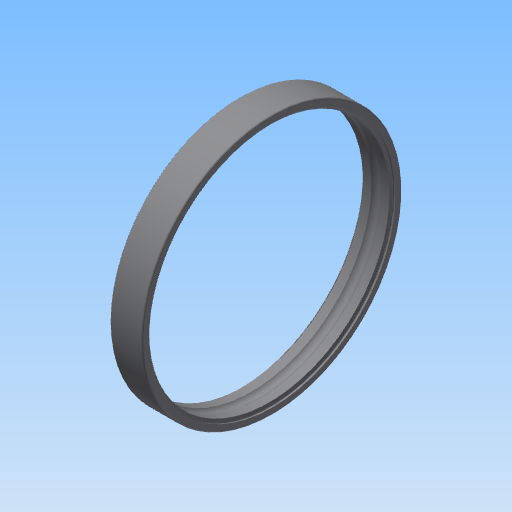
# Autodesk Inventor part: W 61705-2RS1_PART2
Saved by Autodesk Inventor 2021 (Build 250183000, 183)
## iProperties
Category: PARTsolutions
Company: SKF
Created: 2020-02-16
Part Number: W 61705-2RS1_PART2
Material: Allgemein
Catalog Web Link: www.cadenas.de
Description: -Deep groove ball bearings
Vendor: SKF
Document SubType Name: Modeling
Designer: psadmin
Manufacturer: SKF
Mass: 0.422448 g
Surface Area: 10.2422 cm^2
Volume: 0.422448 cm^3
Density: 1 g/cm^3
Appearance: PSOLRGB-175-175-175
PSOL_IDENT_0: {$CADENAS_DATA\23d-libs\skf\bearings_units_and_housings\ball_bearings\deep_groove_ball_bearings\bb1_
PSOL_IDENT_1: 001_101.prj},203 {VTYP=3D},{NB=W 61705-2RS1_PART2},{LINA=W 61705-2RS1_PART2},{NN=BB1_001_101_PART2},
PSOL_IDENT_2: {NOPRJ=TRUE},{DATE=19.12.2019 14:34:47},{GEOMDATE=18.12.2019 13:53:11},{VERSION=},{LINEID=17460},{WB
PSOL_IDENT_3: VAR=},{WBNUMERIC=}  {NB=W 61705-2RS1_PART2},{LINA=W 61705-2RS1_PART2},{KT=DUMMY},{PRODUCTID=},{DESIG
PSOL_IDENT_4: NATION=W 61705-2RS1},{DD=25.000},{D=32.000},{B=4.000},{C=0.000},{DD1=27.35},{DD2=0.00},{D1=0.00},{D2=
PSOL_IDENT_5: 30.29},{D3=0.000},{D4=0.000},{HH=MIN},{BB=0.000},{FF=0.00},{R0MAX=MIN},{R0=MIN},{R12=0.20},{PITCH=28
PSOL_IDENT_6: .50},{DW=1.588},{DDAMIN=26.500},{DDAMAX=27.000},{DDBMIN=MIN},{DDBMAX=MIN},{DBMIN=MIN},{DAMAX=31.000}
PSOL_IDENT_7: ,{BBAMIN=MIN},{CAMAX=MIN},{RAMAX=0.200},{LOAD1=0.618},{LOAD2=0.465},{LOAD3=0.020},{SPEED1=MIN},{SPEE
PSOL_IDENT_8: D2=12000},{KR=0.015},{F0=8.800},{Z=21},{II=1},{MASS=0.007},{BEARING=W 61705-2RS1},{RING=},{HELP=1.21
PSOL_IDENT_9: 8},{HELP2=0.855},{DD1ALG=13.675},{YALG=13.675},{PITCH1=28.500},{DW1=1.588},{YALG1=14.782},{HALG1=1.2
PSOL_IDENT_10: 18},{SH=13.675},{CU=0.482},{DESIGN=dgbbw2rs},{HALG=1.175},{B1=0},{SHIELDHELP=2}
NT: Deep groove ball bearings
NB: W 61705-2RS1_PART2
NBSYN: $DESIGNATION._PART2
LINA: W 61705-2RS1_PART2
SUPPLIER: SKF
ARTICLENO: W 61705-2RS1_PART2
BOMINFO: W 61705-2RS1_PART2
CREATOR: CADENAS GmbH
Title: W 61705-2RS1_PART2
Author: Cadenas PARTsolutions
Comments: Deep groove ball bearings
Autodesk Inventor part; units mm, degrees
ref_plane "YZ Plane" through (0, 0, 0) normal (1, 0, 0) x (0, 1, 0)
ref_plane "XZ Plane" through (0, 0, 0) normal (0, 1, 0) x (-1, 0, 0)
ref_plane "XY Plane" through (0, 0, 0) normal (0, 0, 1) x (1, 0, 0)
sketch "Sketch_16" plane through (0, 0, 0) normal (0, 0, 1) x (1, 0, 0)
  line L0 (50, 0) -> (-50, 0)
  line L1 (0, 15.145) -> (0.06, 15.145)
  arc A0 (0.3, 15.145) -> (0.06, 15.145) centre (0.18, 15.145) ccw
  line L2 (0.3, 15.145) -> (0.364, 14.782)
  line L3 (0.364, 14.782) -> (1.4106, 14.782)
  arc A1 (2.5894, 14.782) -> (1.4106, 14.782) centre (2, 14.25) ccw
  line L4 (2.5894, 14.782) -> (3.636, 14.782)
  line L5 (3.636, 14.782) -> (3.7, 15.145)
  arc A2 (3.94, 15.145) -> (3.7, 15.145) centre (3.82, 15.145) ccw
  line L6 (3.94, 15.145) -> (4, 15.145)
  line L7 (4, 15.145) -> (4, 15.8)
  arc A3 (4, 15.8) -> (3.8, 16) centre (3.8, 15.8) ccw
  line L8 (3.8, 16) -> (0.2, 16)
  arc A4 (0.2, 16) -> (0, 15.8) centre (0.2, 15.8) ccw
  line L9 (0, 15.8) -> (0, 15.145)
  constraints: 20 end point, 10 point on circle, 5 centre point
revolve "Revolution1" add sketch "Sketch_16" angle 360 about axis through (50, 0, 0) along (1, 0, 0)
body "Solid1"
